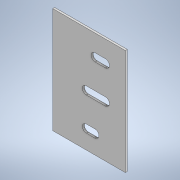
# Autodesk Inventor part: adjust_sheet
Saved by Autodesk Inventor 2021 (Build 250183000, 183)
## iProperties
Created: 2021-06-23
Part Number: adjust_sheet
Material: Generic
Document SubType Name: Modeling
Density: 1 g/cm^3
Appearance: Default
Autodesk Inventor part; units mm, degrees
ref_plane "YZ Plane" through (0, 0, 0) normal (1, 0, 0) x (0, 1, 0)
ref_plane "XZ Plane" through (0, 0, 0) normal (0, 1, 0) x (-1, 0, 0)
ref_plane "XY Plane" through (0, 0, 0) normal (0, 0, 1) x (1, 0, 0)
sketch "Sketch1" plane through (0, 0, 0) normal (0, 0, 1) x (1, 0, 0)
  line L0 (0, 0) -> (-110, 0)
  line L1 (-110, 0) -> (-110, 160)
  line L2 (-110, 160) -> (0, 160)
  line L3 (0, 160) -> (0, 0)
  circle A0 centre (1005.7886, -227) radius 1095
  line L4 (-30, 131.0024) -> (-30, 16.3048)
  line L5 (-45.8188, 136.6478) -> (-45.8188, 11.3835)
  line L6 (-59.0579, 23.7454) -> (-59.0579, 132.6546)
  line L7 (-31.1808, 128.2) -> (-132.5085, 128.2)
  line L8 (-12.6212, 78.2) -> (-114.0631, 78.2)
  line L9 (-53.2816, 28.2) -> (-117.4673, 28.2)
  point P0 (-30, 128.2)
  point P1 (-45.8188, 78.2)
  point P2 (-59.0579, 28.2)
  point P3 (-45.8188, 128.2)
  point P4 (-30, 78.2)
  point P5 (-45.8188, 28.2)
  point P6 (-59.0579, 78.2)
  point P7 (-59.0579, 78.2)
  dimension "d0" = 110
  dimension "d1" = 160
  dimension "d4" = 2190
  dimension "d7" = 30
  dimension "d10" = 50
  dimension "d11" = 50
  dimension "d21" = 305.2
  dimension "d22" = 227
  constraints: 20 end point, 13 point on line, 4 horizontal, 3 point on circle, 3 vertical, 2 parallel, 1 centre point, 1 coincident, 1 midpoint, 1 perpendicular
  measures "d0" distance of L1.end L2.end
  measures "d1" distance between parallel lines of L0 L2
  measures "d4" diameter of A0
  measures "d7" distance from line of L3 A0.start
  measures "d10" distance between parallel lines of L7 L8
  measures "d11" distance between parallel lines of L9 L8
  measures "d21" vertical distance of A0.centre A0.end
  measures "d22" distance from line of L0 A0.centre
extrude "Extrusion1" add sketch "Sketch1" along normal blind 3 contours L0 A0 L8 L4 L2 L3 | L0 L1 L9 A0 | L6 L8 A0 | L9 L1 L8 L6 | A0 L5 L7 L1 L2 | L8 L6 L7 L5 | A0 L4 L8 | L8 L1 L7 L6
hole "Hole1" at (-30, 128.2, 0) at (-45.8188, 78.2, 0) at (-59.0579, 28.2, 0) at (-45.8188, 128.2, 0) at (-30, 78.2, 0) at (-45.8188, 28.2, 0) at (-59.0579, 78.2, 0) direction (0, 0, 1) diameter 12 end through all
sketch "Sketch2" plane through (0, 0, 0) normal (0, 0, -1) x (-1, 0, 0)
  circle A0 centre (30, 128.2) radius 6 projected
  circle A1 centre (45.8188, 128.2) radius 6 projected
  line L0 (30, 122.2) -> (45.8188, 122.2)
  circle A2 centre (30, 128.2) radius 6 projected
  line L1 (30, 134.2) -> (45.8188, 134.2)
  line L2 (30, 134.2) -> (30, 122.2)
  line L3 (45.8188, 122.2) -> (45.8188, 134.2)
  line L4 (30, 84.2) -> (59.0579, 84.2)
  line L5 (30, 72.2) -> (59.0579, 72.2)
  circle A3 centre (30, 78.2) radius 6 projected
  circle A4 centre (59.0579, 78.2) radius 6 projected
  line L6 (30, 84.2) -> (30, 72.2)
  line L7 (59.0579, 72.2) -> (59.0579, 84.2)
  line L8 (45.8188, 34.2) -> (59.0579, 34.2)
  line L9 (45.8188, 22.2) -> (59.0579, 22.2)
  circle A5 centre (45.8188, 28.2) radius 6 projected
  circle A6 centre (59.0579, 28.2) radius 6 projected
  line L10 (45.8188, 22.2) -> (45.8188, 34.2)
  line L11 (59.0579, 22.2) -> (59.0579, 34.2)
  point P0 (0, 0)
  constraints: 24 end point, 10 point on circle, 8 horizontal, 4 tangent, 3 parallel, 3 vertical, 1 vertical alignment, 3 other
extrude "Extrusion2" cut sketch "Sketch2" against normal blind 3 contours A0 L1 A1 L0 | L4 A4 L5 A3 | L8 A6 L9 A5
equation "\"d11\" = d10"
body "Solid1"
